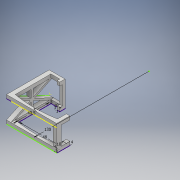
# Autodesk Inventor part: StrumClip1
Saved by Autodesk Inventor 2019 (Build 230136000, 136)
## iProperties
Created: 2017-12-03
Part Number: StrumClip1
Material: Generic
Document SubType Name: Modeling
Designer: Max
Density: 1 g/cm^3
Appearance: Default
Author: Max
Autodesk Inventor part; units mm, degrees
ref_plane "YZ Plane" through (0, 0, 0) normal (1, 0, 0) x (0, 1, 0)
ref_plane "XZ Plane" through (0, 0, 0) normal (0, 1, 0) x (-1, 0, 0)
ref_plane "XY Plane" through (0, 0, 0) normal (0, 0, 1) x (1, 0, 0)
sketch "Sketch1" plane through (0, 0, 0) normal (0, 0, 1) x (1, 0, 0)
  line L0 (0, 0) -> (0, 40.5)
  line L1 (0, 40.5) -> (10, 40.5)
  line L2 (13, 43.5) -> (8, 43.5)
  line L3 (10, 37.5) -> (13, 37.5)
  line L4 (13, 37.5) -> (13, 43.5)
  line L5 (8, 43.5) -> (-5, 43.5)
  line L6 (-5, 43.5) -> (-5, -5)
  line L7 (-5, -5) -> (52, -5)
  line L8 (10, 40.5) -> (10, 37.5)
  line L9 (48, 0) -> (48, 10)
  line L10 (48, 10) -> (52, 10)
  line L11 (52, 10) -> (52, -5)
  arc A0 (0, 0) -> (48, 0) centre (24, 127.7654) ccw
  dimension "d0" = 40.5
  dimension "d2" = 3
  dimension "d7" = 5
  dimension "d8" = 3
  dimension "d9" = 10
  dimension "d10" = 3
  dimension "d20" = 10
  dimension "d23" = 4
  dimension "d24" = 48
  dimension "d25" = 130
  dimension "d26" = 5
  constraints: 24 end point, 4 perpendicular, 4 vertical, 2 horizontal, 2 parallel, 2 point on circle, 1 centre point
  measures "d0" distance of L0.start L0.end
  measures "d2" distance of L3.end L3.start
  measures "d7" distance between parallel lines of L6 L0
  measures "d8" distance between parallel lines of L3 L1
  measures "d9" distance of L0.end L1.end
  measures "d10" distance between parallel lines of L5 L1
  measures "d20" distance of L9.start L9.end
  measures "d23" distance of L9.end L10.end
  measures "d24" distance between parallel lines of L0 L9
  measures "d25" radius of A0
  measures "d26" vertical distance of L9.start L7.end
extrude "Extrusion1" add sketch "Sketch1" along normal blind 4
pattern_linear "Rectangular Pattern1" count 2 spacing 25 along (0, 0, 1) of "Extrusion1"
sketch "Sketch2" plane through (0, 0, 4) normal (0, 0, 1) x (1, 0, 0)
  line L0 (-5, 43.5) -> (-5, -5) projected
  line L1 (-5, -5) -> (0, -5)
  line L2 (0, -5) -> (0, 0)
  line L3 (0, 0) -> (-5, 0)
  line L4 (-5, 0) -> (-5, -5)
  constraints: 8 end point, 2 parallel, 1 horizontal, 1 perpendicular
sketch "Sketch3" plane through (0, 0, 25) normal (1, 0, 0) x (0, 0, -1)
  line L0 (25, 0) -> (21, 0) projected
  line L1 (21, 0) -> (0, 43.5)
  constraints: 2 end point
sweep "Sweep1" add profiles "Sketch2" path "Sketch3" keep normal constant yes
sketch "Sketch4" plane through (52, -5, 25) normal (0, 0, -1) x (-1, 0, 0)
  line L0 (52, 5) -> (52, 0) projected
  line L1 (57, 0) -> (0, 0) projected
  line L2 (52, 5) -> (57, 5)
  line L3 (57, 5) -> (57, 0)
  line L4 (57, 0) -> (52, 0)
  line L5 (52, 0) -> (52, 5)
  constraints: 8 end point, 2 parallel, 1 horizontal, 1 perpendicular
sketch "Sketch5" plane through (-5, -5, 0) normal (-1, 0, 0) x (0, 0, 1)
  line L0 (4, 48.5) -> (25, 5)
  point P0 (0, 5)
  constraints: 2 end point
sweep "Sweep2" add profiles "Sketch4" path "Sketch5"
sketch "Sketch6" plane through (0, 0, 4) normal (0, 0, 1) x (1, 0, 0)
  line L0 (0, 0) -> (0, 40.5) projected
  line L1 (-5, 38.5) -> (-5, 0) projected
  line L2 (0, 18) -> (-5, 18)
  line L3 (-5, 18) -> (-5, 20.5)
  line L4 (-5, 20.5) -> (0, 20.5)
  line L5 (0, 20.5) -> (0, 18)
  line L6 (13, 43.5) -> (10, 43.5)
  line L7 (10, 43.5) -> (10, 40.5)
  line L8 (10, 40.5) -> (13, 40.5)
  line L9 (13, 40.5) -> (13, 43.5)
  line L10 (52, -5) -> (52, 10) projected
  line L11 (48, 10) -> (48, 0) projected
  line L12 (52, -5) -> (48, -5)
  line L13 (48, -5) -> (48, 0)
  line L14 (48, 0) -> (52, 0)
  line L15 (52, 0) -> (52, -5)
  point P0 (-5, 43.5)
  dimension "d27" = 18
  dimension "d28" = 18
  constraints: 24 end point, 6 parallel, 3 horizontal, 3 perpendicular, 2 point on line
  measures "d27" distance from line of L0.start L2
  measures "d28" distance from line of L1.start L4
extrude "Extrusion2" add sketch "Sketch6" along normal blind 21
body "Solid1"
